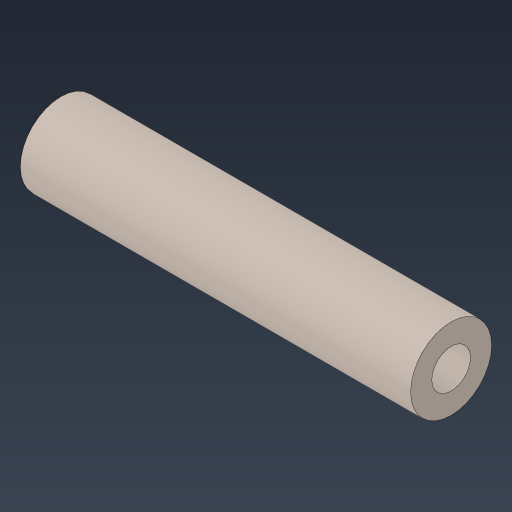
# Autodesk Inventor part: Dribblerschnecke v2
Saved by Autodesk Inventor 2023.1 (Build 271208000, 208)
## iProperties
Part Number: Dribblerschnecke v2
Material: Gummi, Silikon
Document SubType Name: Modeling
Designer: rYan
Mass: 4.63481 g
Surface Area: 37.5203 cm^2
Volume: 3.70785 cm^3
Density: 1.25 g/cm^3
Appearance: Gummi - Schwarz(3)
Author: rYan
Autodesk Inventor part; units mm, degrees
ref_plane "YZ Plane" through (0, 0, 0) normal (1, 0, 0) x (0, 1, 0)
ref_plane "XZ Plane" through (0, 0, 0) normal (0, 1, 0) x (-1, 0, 0)
ref_plane "XY Plane" through (0, 0, 0) normal (0, 0, 1) x (1, 0, 0)
sketch "Skizze1" plane through (0, 0, 0) normal (1, 0, 0) x (0, 1, 0)
  circle A0 centre (0, 0) radius 3.35
  circle A1 centre (0, 0) radius 7
  dimension "d0" = 6.7
  dimension "d1" = 14
  constraints: 2 centre point, 2 coincident
  measures "d0" diameter of A0
  measures "d1" diameter of A1
extrude "Extrusion1" add sketch "Skizze1" along normal blind 33.7
sketch "Skizze3" plane through (0, 0, 0) normal (0, 1, 0) x (-1, 0, 0)
  line L0 (-33.7, 7) -> (-29.7, 7)
  line L1 (-29.7, 7) -> (-29.8763, 8)
  line L2 (-29.8763, 8) -> (-33.7, 7)
  line L3 (-33.7, 7) -> (-33.7, -7) construction
  line L4 (0, -7) -> (0, 7) construction
  line L5 (-36.7, 7) -> (-36.8763, 8) construction
  circle A0 centre (-33.6009, 29.249) radius 21.5 construction
  line L6 (-28.161, 8.4486) -> (-33.6009, 29.249) construction
  line L7 (-29.8763, 8) -> (-36.8763, 8) construction
  point P0 (0, 0)
  dimension "d98" = 43
  dimension "d16" = 4
  dimension "d17" = 80
  dimension "d18" = 1
  dimension "d96" = 7
  dimension "d126" = 14.656
  constraints: 12 end point, 2 horizontal, 2 point on line, 1 coincident, 1 parallel, 1 perpendicular, 4 other
  measures "d16" distance of L0.start L0.end
  measures "d17" angle of L1 L0
  measures "d18" distance from line of L0 L1.end
  measures "d96" distance of L5.start L0.end
  measures "d126" angle of L0 L2
feature "Spirale1" [suppressed]
sketch "Skizze20" plane through (18.7, -3.5355, -3.5355) normal (0, 0.7071068, -0.7071068) x (1, 0, 0)
  line L0 (4, 0) -> (0, 0) projected
  line L1 (4, 0) -> (0.1763, 1) projected
  line L2 (0.1763, 1) -> (0, 0) projected
  point P0 (-18.7, -5)
feature "Spirale3" [suppressed]
sketch "Skizze24" plane through (10.7739, 3.0836, -3.9359) normal (0, 0.7871835, 0.6167189) x (1, 0, 0)
  line L0 (2.323, 0) -> (0, 0) projected
  line L1 (2.323, 0) -> (0.1024, 0.5807) projected
  line L2 (0.1024, 0.5807) -> (0, 0) projected
  point P0 (-10.7739, -5)
feature "Spirale4" [suppressed]
mirror "Spiegeln2" about plane through (0, 0, 0) normal (1, 0, 0) of "Extrusion1"
sketch "Skizze25" plane through (2.8479, -4.8082, 1.3717) normal (0, -0.2743466, -0.9616309) x (1, 0, 0)
  circle A0 centre (-2.8479, 21.4682) radius 21.5
  circle A1 centre (1.449, 21.6145) radius 21.5
  circle A2 centre (13.3899, 22.0495) radius 21.5
  point P0 (-2.8479, -5)
  point P1 (-5.7242, 0.1615)
  point P2 (0.0285, 0.1615)
  dimension "d163" = 43
  dimension "d162" = 43
  dimension "d164" = 43
  constraints: 2 centre point, 2 point on circle, 3 other
  measures "d162" diameter of A0
  measures "d164" diameter of A2
sketch "Skizze26" plane through (0, 0, 0) normal (0, 0, 1) x (1, 0, 0)
  line L0 (-33.7, -7) -> (-33.7, 7) construction
  line L1 (33.7, -7) -> (33.7, 7) construction
  arc A0 (-33.7, 7) -> (33.7, 7) centre (0, 574.345) ccw
  line L2 (-33.7, 6) -> (33.7, 6) construction
  line L3 (-33.7, 7) -> (33.7, 7)
  line L4 (-33.7, 0) -> (33.7, 0)
  point P0 (0, 0)
  dimension "d165" = 1
  constraints: 6 end point, 2 midpoint, 2 perpendicular, 2 point on circle, 2 point on line, 1 centre point, 1 tangent
  measures "d165" distance between parallel lines of L3 L2
revolve "Umdrehung5" [suppressed]
